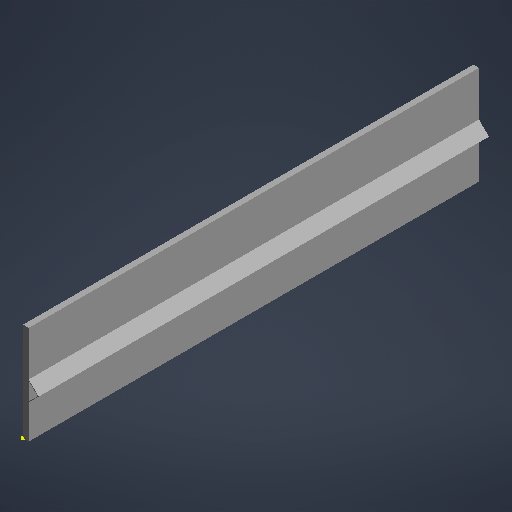
# Autodesk Inventor part: Riel Inferior
Saved by Autodesk Inventor 2026.2 (Build 302298010, 298A)
## iProperties
Part Number: Riel Inferior
Material: Generic
Document SubType Name: Modeling
Designer: diego
Appearance: Default
Author: diego
Autodesk Inventor part; units mm, degrees
ref_plane "YZ Plane" through (0, 0, 0) normal (1, 0, 0) x (0, 1, 0)
ref_plane "XZ Plane" through (0, 0, 0) normal (0, 1, 0) x (-1, 0, 0)
ref_plane "XY Plane" through (0, 0, 0) normal (0, 0, 1) x (1, 0, 0)
sketch "Sketch1" plane through (0, 0, 0) normal (1, 0, 0) x (0, 1, 0)
  point P0 (0, 0)
sketch "Sketch2" plane through (0, 0, 0) normal (1, 0, 0) x (0, 1, 0)
  line L0 (0, 0) -> (350, 0)
  line L1 (350, 0) -> (350, -1600)
  line L2 (350, -1600) -> (0, -1600)
  line L3 (0, -1600) -> (0, 0)
  dimension "d0" = 350
  dimension "d1" = 1600
  constraints: 8 end point, 2 parallel, 1 horizontal, 1 perpendicular
  measures "d0" distance of L1.end L2.end
  measures "d1" distance of L0.end L1.end
extrude "Extrusion1" add sketch "Sketch2" along normal blind 20
sketch "Sketch5" plane through (0, 0, 0) normal (0, 0, 1) x (1, 0, 0)
  line L0 (20, 0) -> (20, 350) projected
  line L1 (20, 191.3422) -> (55.3553, 155.9868)
  line L2 (20, 191.3422) -> (70, 191.3422) construction
  line L3 (55.3553, 155.9868) -> (20, 120.6315)
  line L4 (20, 120.6315) -> (20, 123.4764)
  line L5 (20, 123.4764) -> (52.1099, 155.5863)
  line L6 (52.1099, 155.5863) -> (20, 187.6962)
  line L7 (20, 187.6962) -> (20, 191.3422)
  point P0 (0, 0)
  dimension "d10" = 50
  dimension "d11" = 45
  dimension "d12" = 50
  constraints: 14 end point, 4 point on line, 1 collinear, 1 equal length, 1 horizontal, 1 parallel, 1 perpendicular
  measures "d10" distance of L1.start L1.end
  measures "d11" angle of L1 L2
  measures "d12" distance of L1.end L3.end
extrude "Extrusion3" add sketch "Sketch5" against normal blind 1600 contours L0 L5 L6 L1 L3
body "Solid1"
